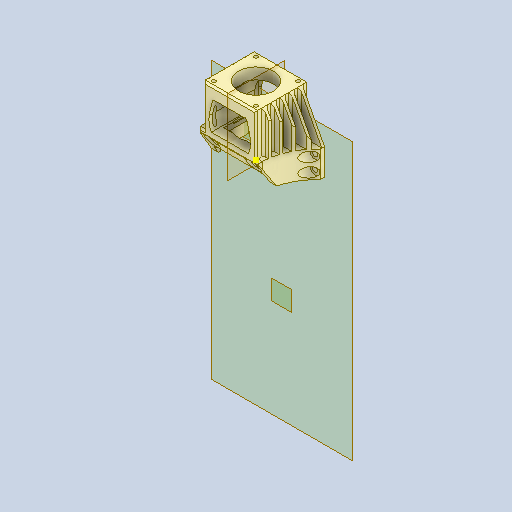
# Autodesk Inventor part: Z_Motor_Holder
Saved by Autodesk Inventor 2023 (Build 270158000, 158)
## iProperties
Created: 2022-09-04
Part Number: Z_Motor_Holder
Material: Nylon, molybdenum disulphide
Document SubType Name: Modeling
Designer: plebbb
Density: 1.13 g/cm^3
Appearance: Nylon 6
Author: plebbb
Autodesk Inventor part; units mm, degrees
ref_plane "YZ Plane" through (0, 0, 0) normal (1, 0, 0) x (0, 1, 0)
ref_plane "XZ Plane" through (0, 0, 0) normal (0, 1, 0) x (-1, 0, 0)
ref_plane "XY Plane" through (0, 0, 0) normal (0, 0, 1) x (1, 0, 0)
sketch "Sketch1" plane through (0, 0, 0) normal (0, 1, 0) x (-1, 0, 0)
  line L0 (0, 0) -> (58.4, 0)
  line L1 (58.4, 0) -> (58.4, -58.4)
  line L2 (58.4, -58.4) -> (0, -58.4)
  line L3 (0, -58.4) -> (0, 0)
  circle A0 centre (29.2, -29.2) radius 19.3
  circle A1 centre (5.63, -5.63) radius 2.1
  circle A2 centre (52.77, -52.77) radius 2.1
  circle A3 centre (5.63, -52.77) radius 2.1
  circle A4 centre (52.77, -5.63) radius 2.1
  line L4 (52.77, -5.63) -> (5.63, -5.63) construction
  line L5 (5.63, -5.63) -> (5.63, -52.77) construction
  line L6 (5.63, -52.77) -> (52.77, -52.77) construction
  line L7 (52.77, -52.77) -> (52.77, -5.63) construction
  point P0 (58.4, -29.2)
  point P1 (29.2, -58.4)
  point P2 (29.2, -52.77)
  point P3 (52.77, -29.2)
  dimension "d2" = 58.4
  dimension "d3" = 38.6
  dimension "d4" = 47.14
  dimension "d5" = 4.2
  constraints: 16 end point, 5 centre point, 4 coincident, 4 midpoint, 4 parallel, 4 perpendicular, 3 equal radius, 2 horizontal, 2 horizontal alignment, 2 vertical alignment
  measures "d2" distance of L0.end L1.end
  measures "d3" diameter of A0
  measures "d4" distance of L6.end L4.start
  measures "d5" diameter of A4
extrude "Extrusion1" add sketch "Sketch1" along normal blind 7.5
sketch "Sketch2" plane through (-58.4, 0, 0) normal (0, 0, 1) x (1, 0, 0)
  line L0 (0, 0) -> (58.4, 0) projected
  line L1 (0, 0) -> (58.4, 0)
  line L2 (58.4, 0) -> (58.4, -39.35)
  line L3 (58.4, -39.35) -> (0, -39.35)
  line L4 (0, -39.35) -> (0, 0)
  line L5 (12.1029, -5) -> (46.2971, -5)
  arc A0 (12.1029, -5) -> (10.2, -6.3844) centre (12.1029, -7) ccw
  arc A1 (48.2, -6.3844) -> (46.2971, -5) centre (46.2971, -7) ccw
  arc A2 (10.2, -6.3844) -> (5, -39.35) centre (112.0936, -39.35) ccw
  arc A3 (53.4, -39.35) -> (48.2, -6.3844) centre (-53.6936, -39.35) ccw
  line L6 (-41.8, -39.85) -> (100.2, -39.85) construction
  arc A4 (6.308, -22.6634) -> (10, -39.35) centre (29.3999, -26.3059) ccw
  arc A5 (48.4, -39.35) -> (52.092, -22.6634) centre (29.0001, -26.3059) ccw
  line L7 (8.7957, -37.35) -> (49.6043, -37.35)
  point P0 (29.2, -5)
  point P1 (29.2, -39.35)
  point P2 (29.2, 0)
  point P3 (29.2, -37.35)
  dimension "d9" = 2
  dimension "d10" = 5
  dimension "d12" = 5
  dimension "d13" = 38
  dimension "d18" = 0.5
  dimension "d19" = 5
  dimension "d20" = 2
  constraints: 16 point on circle, 12 end point, 6 centre point, 6 tangent, 4 midpoint, 4 point on line, 3 equal radius, 3 horizontal, 2 line through centre, 2 parallel, 1 horizontal alignment, 1 perpendicular, 1 vertical alignment
  measures "d9" radius of A0
  measures "d10" distance of point (29.2, 0) point (29.2, -5)
  measures "d12" distance of A2.end L3.end
  measures "d13" distance of A1.start A0.end
  measures "d18" vertical distance of L6.start L3.end
  measures "d19" distance of A4.end A2.end
  measures "d20" distance of point (29.2, -39.35) point (29.2, -37.35)
extrude "Extrusion2" add sketch "Sketch2" against normal up to surface (58.4 mm away) contours L0 L2 L3 A3 A1 L5 A0 A2 L4 | A2 A4 L3 | L3 A5 A3 | A4 L7 A5 L3
sketch "Sketch3" plane through (0, 7.5, 0) normal (0, 1, 0) x (1, 0, 0)
  circle A0 centre (-52.77, 5.63) radius 2.1 projected
  circle A1 centre (-5.63, 5.63) radius 2.1 projected
  circle A2 centre (-52.77, 52.77) radius 2.1 projected
  circle A3 centre (-5.63, 52.77) radius 2.1 projected
  circle A4 centre (-29.2, 29.2) radius 19.3 projected
  point P0 (0, 0)
extrude "Extrusion3" cut sketch "Sketch3" against normal up to surface (46.85 mm away)
sketch "Sketch4" plane through (-58.4, -39.35, 0) normal (0, -1, 0) x (1, 0, 0)
  line L0 (39.0137, -30.7) -> (39.0137, -27.7) projected
  line L1 (39.0137, -27.7) -> (30.7, -19.3863) projected
  line L2 (30.7, -19.3863) -> (27.7, -19.3863) projected
  line L3 (27.7, -19.3863) -> (19.3863, -27.7) projected
  line L4 (19.3863, -27.7) -> (19.3863, -30.7) projected
  line L5 (19.3863, -30.7) -> (27.7, -39.0137) projected
  line L6 (27.7, -39.0137) -> (30.7, -39.0137) projected
  line L7 (30.7, -39.0137) -> (39.0137, -30.7) projected
  line L8 (46.2, -12.2) -> (46.2, -46.2) projected
  line L9 (46.2, -46.2) -> (12.2, -46.2) projected
  line L10 (12.2, -46.2) -> (12.2, -12.2) projected
  line L11 (12.2, -12.2) -> (46.2, -12.2) projected
  line L12 (11.2, -47.2) -> (47.2, -47.2)
  line L13 (47.2, -47.2) -> (47.2, -11.2)
  line L14 (47.2, -11.2) -> (11.2, -11.2)
  line L15 (11.2, -11.2) -> (11.2, -47.2)
  line L16 (-41.8, -51.2) -> (100.2, -51.2) projected
  line L17 (-5, -51.2) -> (63.4, -51.2)
  line L18 (63.4, -51.2) -> (63.4, 0)
  line L19 (63.4, 0) -> (-5, 0)
  line L20 (-5, 0) -> (-5, -51.2)
  line L21 (0, 0) -> (58.4, 0) projected
  line L22 (0, 0) -> (0, -58.4) projected
  line L23 (58.4, 0) -> (58.4, -58.4) projected
  dimension "d21" = 1
  dimension "d22" = 1
  dimension "d23" = 1
  dimension "d24" = 0
  dimension "d25" = 5
  dimension "d26" = 5
  constraints: 16 end point, 4 perpendicular, 3 parallel, 1 collinear, 1 horizontal, 1 point on line
  measures "d21" distance between parallel lines of L10 L15
  measures "d22" distance between parallel lines of L14 L11
  measures "d23" distance between parallel lines of L12 L9
  measures "d24" distance between parallel lines of L16 L17
  measures "d25" distance between parallel lines of L18 L23
  measures "d26" distance between parallel lines of L20 L22
extrude "Extrusion4" add sketch "Sketch4" along normal blind 4.35 contours L20 L19 L22 L16 | L22 L19 L23 L16 | L23 L19 L18 L16
sketch "Sketch5" plane through (-58.4, -43.7, 0) normal (0, -1, 0) x (1, 0, 0)
  line L0 (11.2, -47.2) -> (11.2, -11.2) projected
  line L1 (11.2, -11.2) -> (47.2, -11.2) projected
  line L2 (47.2, -11.2) -> (47.2, -47.2) projected
  line L3 (47.2, -47.2) -> (11.2, -47.2) projected
  point P0 (58.4, 0)
extrude "Extrusion5" cut sketch "Sketch5" against normal blind 10.1
sketch "Sketch6" plane through (-63.4, -39.35, -51.2) normal (-1, 0, 0) x (0, 0, 1)
  line L0 (51.2, -4.35) -> (0, -4.35) projected
  line L1 (0, -4.35) -> (0, -29.5)
  line L2 (32.5, -29.5) -> (32.5, -4.5) projected
  line L3 (40, -4.35) -> (4, -4.35) projected
  line L4 (32.65, -4.35) -> (32.65, -29.5)
  line L5 (32.65, -29.5) -> (35.15, -29.5)
  line L6 (35.15, -29.5) -> (51.2, -4.35)
  point P0 (51.2, 39.35)
  point P1 (38.75, -29.5)
  dimension "d31" = 0.15
  dimension "d32" = 2.5
  constraints: 8 end point, 2 horizontal alignment, 1 horizontal, 1 perpendicular, 1 point on line, 1 vertical, 1 other
  measures "d31" distance between parallel lines of L4 L2
  measures "d32" distance of L4.end L5.end
extrude "Extrusion6" add sketch "Sketch6" against normal up to surface (68.4 mm away)
sketch "Sketch7" plane through (-63.4, -39.35, -51.2) normal (-1, 0, 0) x (0, 0, 1)
  line L0 (4, -4.35) -> (32.65, -4.35) projected
  line L1 (32.65, -4.35) -> (0, -4.35)
  line L2 (0, -4.35) -> (0, -29.5)
  line L3 (0, -29.5) -> (32.65, -29.5)
  line L4 (32.65, -29.5) -> (32.65, -4.35)
  point P0 (51.2, 39.35)
  constraints: 8 end point, 2 parallel, 1 coincident, 1 horizontal, 1 perpendicular
extrude "Extrusion7" add sketch "Sketch7" against normal blind 4
ref_plane "Work Plane1" through (-29.2, 7.5, 0) normal (1, 0, 0) x (0, 0, -1)
mirror "Mirror1" about plane through (-29.2, 7.5, 0) normal (1, 0, 0) of "Extrusion7"
sketch "Sketch8" plane through (5, -68.85, -51.2) normal (0, -1, 0) x (1, 0, 0)
  line L0 (-51.2, 39) -> (-17.2, 39) projected
  line L1 (-51.2, 32.5) -> (-51.2, 39) projected
  line L2 (-17.2, 39) -> (-17.2, 32.5) projected
  line L3 (-51.5, 39.3) -> (-16.9, 39.3)
  line L4 (-16.9, 39.3) -> (-16.9, 32.5)
  line L5 (-16.9, 32.5) -> (-51.5, 32.5)
  line L6 (-51.5, 32.5) -> (-51.5, 39.3)
  point P0 (-5, 51.2)
  point P1 (-17.2, 35.75)
  point P2 (-17.2, 32.5)
  dimension "d37" = 0.3
  dimension "d38" = 0.3
  dimension "d39" = 0.3
  constraints: 8 end point, 2 parallel, 1 horizontal, 1 midpoint, 1 perpendicular, 1 point on line
  measures "d37" distance between parallel lines of L0 L3
  measures "d38" distance between parallel lines of L6 L1
  measures "d39" distance from line of point (-17.2, 35.75) L4
extrude "Extrusion8" cut sketch "Sketch8" against normal up to surface (31.5 mm away) contours L0 L2 L5 L1
sketch "Sketch10" plane through (-58.4, -39.35, 0) normal (0, 1, 0) x (1, 0, 0)
  line L0 (-5, 0) -> (-5, 51.2) projected
  line L1 (-5, 51.2) -> (-25, 51.2)
  line L2 (-25, 51.2) -> (-25, 46.2)
  arc A0 (-5, 0) -> (-25, 46.2) centre (-68.361, 0) ccw
  point P0 (58.4, 0)
  dimension "d42" = 20
  dimension "d43" = 5
  constraints: 4 end point, 2 point on circle, 1 centre point, 1 horizontal, 1 perpendicular, 1 tangent
  measures "d42" distance of L0.end L1.end
  measures "d43" distance of L1.end L2.end
extrude "Extrusion9" add sketch "Sketch10" against normal up to surface (29.5 mm away)
sketch "Sketch9" plane through (-58.4, -39.35, 0) normal (0, 1, 0) x (1, 0, 0)
  point P0 (58.4, 0)
sketch "Sketch11" plane through (-63.4, -68.85, 0) normal (1, 0, 0) x (0, 0, -1)
  line L0 (16.05, 0) -> (0, 25.15) projected
  line L1 (0, 25.15) -> (0, 0) projected
  line L2 (0, 0) -> (16.05, 0) projected
  point P0 (0, 68.85)
extrude "Extrusion10" cut sketch "Sketch11" along normal mid plane 217.5
sketch "Sketch12" plane through (5, -39.35, -51.2) normal (0, 0, -1) x (-1, 0, 0)
  circle A0 centre (82.9, -7.25) radius 2.8813
  circle A1 centre (82.9, -22.25) radius 2.8813
  line L0 (88.4, 0) -> (88.4, -29.5) projected
  line L1 (82.9, -7.25) -> (82.9, -22.25) construction
  point P0 (5, 39.35)
  point P1 (82.9, -14.75)
  point P2 (88.4, -14.75)
  dimension "d48" = 5.7625
  dimension "d50" = 5.5
  dimension "d51" = 15
  constraints: 2 centre point, 2 end point, 2 midpoint, 1 equal radius, 1 horizontal alignment, 1 vertical, 1 vertical alignment
  measures "d48" diameter of A0
  measures "d50" distance from line of L0 L1.start
  measures "d51" distance of L1.start L1.end
extrude "Extrusion11" cut sketch "Sketch12" against normal blind 217.5
ref_plane "Work Plane2" through (5, -39.35, -46.2) normal (0, 0, -1) x (-1, 0, 0)
sketch "Sketch13" plane through (5, -39.35, -46.2) normal (0, 0, -1) x (-1, 0, 0)
  circle A0 centre (82.9, -7.25) radius 5.5
  circle A1 centre (82.9, -22.25) radius 5.5
  circle A2 centre (82.9, -7.25) radius 2.8813 projected
  circle A3 centre (82.9, -22.25) radius 2.8813 projected
  point P0 (5, 39.35)
  dimension "d55" = 11
  constraints: 2 centre point, 2 concentric, 1 equal radius
  measures "d55" diameter of A0
extrude "Extrusion12" cut sketch "Sketch13" against normal blind 217.5 contours A0 | A1 | A2 | A3
mirror "Mirror2" about plane through (-29.2, 7.5, 0) normal (1, 0, 0) of "Extrusion12", "Extrusion11", "Extrusion10", "Extrusion9"
sketch "Sketch14" plane through (-7.0247, -39.35, -51.2) normal (0, 0, -1) x (-1, 0, 0)
  line L0 (-7.0247, 0) -> (-32.0247, 0) projected
  line L1 (-7.0247, 0) -> (-7.0247, 46.85) projected
  line L2 (-32.0247, 0) -> (-7.0247, 46.85)
  line L3 (51.3753, 46.85) -> (-7.0247, 46.85) projected
  line L4 (76.3753, 0) -> (51.3753, 0) projected
  line L5 (51.3753, 46.85) -> (76.3753, 0)
  arc A0 (41.1753, 32.9656) -> (39.2724, 34.35) centre (39.2724, 32.35) ccw projected
  arc A1 (45.0673, 16.6866) -> (41.1753, 32.9656) centre (-60.7183, 0) ccw projected
  arc A2 (42.5796, 2) -> (45.0673, 16.6866) centre (21.9754, 13.0441) ccw projected
  line L6 (1.771, 2) -> (42.5796, 2) projected
  arc A3 (-0.7167, 16.6866) -> (1.771, 2) centre (22.3753, 13.0441) ccw projected
  arc A4 (3.1753, 32.9656) -> (-0.7167, 16.6866) centre (105.0689, 0) ccw projected
  arc A5 (5.0782, 34.35) -> (3.1753, 32.9656) centre (5.0782, 32.35) ccw projected
  line L7 (39.2724, 34.35) -> (5.0782, 34.35) projected
  line L8 (51.3753, 0) -> (51.3753, 46.85) projected
  line L9 (-7.0247, 46.85) -> (51.3753, 46.85) projected
  line L10 (-7.0247, 0) -> (-7.0247, 46.85) projected
  line L11 (51.3753, 0) -> (-7.0247, 0) projected
  point P0 (-7.0247, 39.35)
  point P1 (51.3753, 46.85)
  constraints: 4 end point
extrude "Extrusion13" add sketch "Sketch14" against normal blind 3 contours L0 L2 L1 | L8 L5 L4
pattern_linear "Rectangular Pattern1" count 5 spacing 10 along (0, 0, 1) of "Extrusion13"
mirror "Mirror3" about plane through (-29.2, 7.5, 0) normal (1, 0, 0) of "Extrusion13", "Rectangular Pattern1"
sketch "Sketch15" plane through (-59.4, -68.85, -51.2) normal (0, -1, 0) x (1, 0, 0)
  arc A0 (-4.5329, 43) -> (-4, 51.2) centre (-67.361, 51.2) ccw projected
  arc A1 (-6.6702, 33) -> (-4.9977, 40) centre (-67.361, 51.2) ccw projected
  arc A2 (-4.9977, 40) -> (-4.5329, 43) centre (-67.361, 51.2) ccw projected
  arc A3 (-7.6519, 30) -> (-6.6702, 33) centre (-67.361, 51.2) ccw projected
  arc A4 (-10.6215, 23) -> (-7.6519, 30) centre (-67.361, 51.2) ccw projected
  arc A5 (-12.2141, 20) -> (-10.6215, 23) centre (-67.361, 51.2) ccw projected
  arc A6 (-16.8103, 13) -> (-12.2141, 20) centre (-67.361, 51.2) ccw projected
  arc A7 (-19.2239, 10) -> (-16.8103, 13) centre (-67.361, 51.2) ccw projected
  arc A8 (-24, 5) -> (-19.2239, 10) centre (-67.361, 51.2) ccw projected
  line L0 (-4, 51.2) -> (-24, 51.2)
  line L1 (-24, 51.2) -> (-24, 5)
  point P0 (59.4, 51.2)
  constraints: 4 end point, 1 perpendicular, 1 vertical
extrude "Extrusion14" cut sketch "Sketch15" against normal up to surface (76.35 mm away)
mirror "Mirror4" about plane through (-29.2, 7.5, 0) normal (1, 0, 0) of "Extrusion14"
chamfer "Chamfer1" distance 2 angle 45 7 edges at (-58.4, -15.925, 0) (-29.2, 7.5, 0) (0, -15.925, 0) (-60.9, -39.35, 0) (-63.4, -41.525, 0) (2.5, -39.35, 0) (5, -41.525, 0)
fillet "Fillet1" radius 2 3 edges at (-29.2, -43.7, 0) (-58.9, -43.7, 0) (0.5, -43.7, 0)
ref_plane "Work Plane4" through (-29.2, -213.106, -57.7532) normal (0, 0, -1) x (0, -1, 0)
ref_plane "Work Plane5" through (-29.2, -213.106, -57.9032) normal (0, 0, -1) x (0, -1, 0)
sketch "Sketch16" plane through (-29.2, -213.106, -57.9032) normal (0, 0, -1) x (0, -1, 0)
  arc A0 (-206.7216, 19) -> (-208.106, 17.0971) centre (-206.106, 17.0971) ccw projected
  arc A1 (-190.4426, 22.892) -> (-206.7216, 19) centre (-173.756, -82.8936) ccw projected
  arc A2 (-175.756, 20.4043) -> (-190.4426, 22.892) centre (-186.8001, -0.1999) ccw projected
  line L0 (-175.756, -20.4043) -> (-175.756, 20.4043) projected
  arc A3 (-190.4426, -22.892) -> (-175.756, -20.4043) centre (-186.8001, 0.1999) ccw projected
  arc A4 (-206.7216, -19) -> (-190.4426, -22.892) centre (-173.756, 82.8936) ccw projected
  arc A5 (-208.106, -17.0971) -> (-206.7216, -19) centre (-206.106, -17.0971) ccw projected
  line L1 (-208.106, 17.0971) -> (-208.106, -17.0971) projected
  line L2 (-173.756, 29.2) -> (-220.606, 29.2) projected
  line L3 (-220.606, -29.2) -> (-220.606, 29.2) projected
  line L4 (-173.756, -29.2) -> (-220.606, -29.2) projected
  line L5 (-173.756, 29.2) -> (-173.756, -29.2) projected
  line L6 (-220.606, -29.2) -> (-173.756, -29.2) projected
  line L7 (-173.756, -29.2) -> (-163.756, -29.2)
  line L8 (-163.756, -29.2) -> (-163.756, 29.2)
  line L9 (-163.756, 29.2) -> (-173.756, 29.2)
  point P0 (-213.106, -29.2)
  dimension "d69" = 10
  constraints: 6 end point, 2 perpendicular, 1 horizontal
  measures "d69" distance between parallel lines of L5 L8
extrude "Extrusion15" [suppressed]
chamfer "Chamfer2" distance 2 angle 45 24 edges at (0, -15.925, -41.2) (0, -15.925, -51.2) (0, -15.925, -31.2) (0, -15.925, -21.2) (0, -15.925, -11.2) (0, -15.925, -48.2) (0, -15.925, -38.2) (0, -15.925, -28.2) (0, -15.925, -18.2) (0, -15.925, -8.2) (-58.4, -15.925, -8.2) (-58.4, -15.925, -18.2) (-58.4, -15.925, -28.2) (-58.4, -15.925, -38.2) (-58.4, -15.925, -48.2) (-58.4, -15.925, -11.2) (-58.4, -15.925, -21.2) (-58.4, -15.925, -31.2) (-58.4, -15.925, -41.2) (-58.4, -15.925, -51.2) (-58.4, -15.925, -58.4) (0, -15.925, -58.4) (-29.2, 7.5, -58.4) (-29.2, -39.35, -58.4)
sketch "Sketch18" plane through (-56.4, 5.5, 0) normal (0, 0, 1) x (1, 0, 0)
  circle A0 centre (4.2, -68.35) radius 5.4 projected
  circle A1 centre (50.2, -55.35) radius 5.4 projected
  circle A2 centre (50.2, -68.35) radius 5.4 projected
  circle A3 centre (4.2, -55.35) radius 5.4 projected
  circle A4 centre (4.2, -55.35) radius 3.3 projected
  circle A5 centre (4.2, -68.35) radius 3.3 projected
  circle A6 centre (50.2, -68.35) radius 3.3 projected
  circle A7 centre (50.2, -55.35) radius 3.3 projected
  circle A8 centre (50.2, -55.35) radius 3.3 projected
  circle A9 centre (50.2, -68.35) radius 5.6
  circle A10 centre (50.2, -55.35) radius 5.6
  circle A11 centre (4.2, -55.35) radius 5.6
  circle A12 centre (4.2, -68.35) radius 5.6
  point P0 (56.4, -5.5)
  dimension "d78" = 0.2
  constraints: 4 centre point, 4 concentric, 3 equal radius
  measures "d78" radial gap between concentric circles of A11 A3
extrude "Extrusion16" cut sketch "Sketch18" against normal blind 37 contours A0 | A1 | A2 | A3 | A4 | A5 | A6 | A7 | A9 | A10 | A11 | A12
sketch "Sketch21" plane through (-56.4, 5.5, 0) normal (0, 0, 1) x (1, 0, 0)
  line L0 (10.2, -74.35) -> (63.4665, -74.35) projected
  line L1 (-3, -74.35) -> (10.2, -74.35) projected
  line L2 (9.8, -74.35) -> (10.2, -74.35)
  circle A0 centre (50.2, -68.35) radius 5.6 projected
  line L3 (4.2, -62.75) -> (50.2, -62.75)
  line L4 (55.8, -68.35) -> (55.8, -74.35)
  circle A1 centre (4.2, -68.35) radius 5.6 projected
  line L5 (-1.4, -68.35) -> (-1.4, -74.35)
  line L6 (10.2, -74.35) -> (-9.0665, -74.35) projected
  point P0 (56.4, -5.5)
  point P1 (-8.0024, -74.35)
  point P2 (-1.4, -74.35)
  constraints: 8 end point, 4 point on circle, 3 point on line, 2 horizontal, 1 horizontal alignment, 1 perpendicular, 1 vertical, 1 vertical alignment
extrude "Extrusion17" cut sketch "Sketch21" against normal blind 37
chamfer "Chamfer3" distance 2 angle 45 2 edges at (-57.8, -49.85, -3.9248) (-11.8, -49.85, -3.9248)
body "Solid1"
